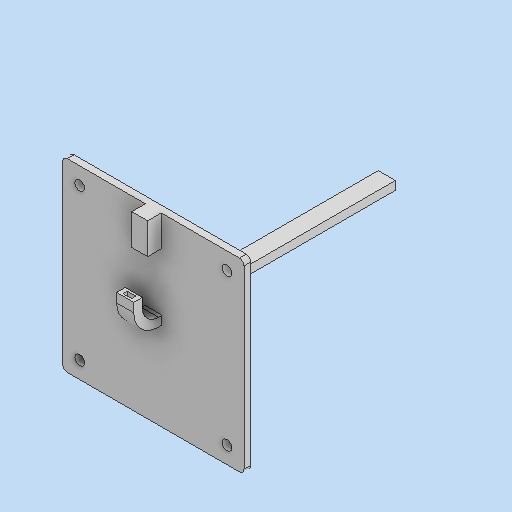
# Autodesk Inventor part: ProbeAntennaDummy
Saved by Autodesk Inventor 2023.2 (Build 272271000, 271)
## iProperties
Created: 2024-02-15
Part Number: ProbeAntennaDummy
Material: Generisch
Document SubType Name: Modeling
Designer: Nils Bade
Density: 1 g/cm^3
Appearance: Vorgabe
Description: Dummy
Auf Bestellliste: True
Author: Nils Bade
Autodesk Inventor part; units mm, degrees
sketch "S-Basis" plane through (0, 0, 0) normal (0, 0, 1) x (1, 0, 0)
  line L0 (0, 57.19) -> (0, -57.19) construction
  line L1 (-56, 0) -> (56, 0) construction
  line L2 (1.8795, -0.94) -> (1.8795, 0.94)
  line L3 (1.8795, 0.94) -> (-1.8795, 0.94)
  line L4 (-1.8795, 0.94) -> (-1.8795, -0.94)
  line L5 (-1.8795, -0.94) -> (1.8795, -0.94)
  line L6 (1.8795, -0.94) -> (-1.8795, 0.94) construction
  line L7 (1.8795, 0.94) -> (-1.8795, -0.94) construction
  line L8 (-40, 40.85) -> (40, 40.85)
  line L9 (40, 40.85) -> (40, -40.85)
  line L10 (40, -40.85) -> (-40, -40.85)
  line L11 (-40, -40.85) -> (-40, 40.85)
  line L12 (-40, 40.85) -> (40, -40.85) construction
  line L13 (40, 40.85) -> (-40, -40.85) construction
  line L14 (-40, 33.35) -> (40, 33.35) construction
  circle A0 centre (0, 33.35) radius 2.5 construction
  line L15 (-40, 13.03) -> (40, 13.03) construction
  line L16 (-3.7747, 1.8879) -> (3.7747, 1.8879)
  line L17 (3.7747, 1.8879) -> (3.7747, -1.8879)
  line L18 (3.7747, -1.8879) -> (-3.7747, -1.8879)
  line L19 (-3.7747, -1.8879) -> (-3.7747, 1.8879)
  line L20 (-3.7747, 1.8879) -> (3.7747, -1.8879) construction
  line L21 (3.7747, 1.8879) -> (-3.7747, -1.8879) construction
  circle A1 centre (-32.5, 33.35) radius 2.15
  circle A2 centre (32.5, 33.35) radius 2.15
  circle A3 centre (-32.5, -33.35) radius 2.15
  circle A4 centre (32.5, -33.35) radius 2.15
  line L22 (-3.5, 40.85) -> (3.5, 40.85)
  line L23 (3.5, 40.85) -> (3.5, 27.1517)
  line L24 (3.5, 27.1517) -> (-3.5, 27.1517)
  line L25 (-3.5, 27.1517) -> (-3.5, 40.85)
  point P0 (0, 0)
  point P1 (0, 40.85)
  dimension "d0" = 81.7
  dimension "d1" = 80
  dimension "d2" = 3.759
  dimension "d3" = 1.88
  dimension "d4" = 7.5
  dimension "d5" = 5
  dimension "d6" = 20.32
  dimension "d7" = 4.3
  dimension "d8" = 32.5
  dimension "d9" = 4.3
  dimension "d10" = 32.5
  dimension "d11" = 7.5
  dimension "d23" = 7
  constraints: 48 end point, 8 midpoint, 8 parallel, 7 point on line, 6 perpendicular, 5 centre point, 4 horizontal, 2 symmetric about line, 2 other
  measures "d0" distance of L8.end L9.end
  measures "d1" distance of L8.start L8.end
  measures "d2" distance of L2.end L3.end
  measures "d3" distance of L2.start L2.end
  measures "d4" distance between parallel lines of L14 L8
  measures "d5" diameter of A0
  measures "d6" distance from line of L15 A0.centre
  measures "d7" diameter of A1
  measures "d8" distance from line of L0 A1.centre
  measures "d9" diameter of A3
  measures "d10" distance from line of L0 A3.centre
  measures "d11" distance from line of L10 A3.centre
  measures "d23" distance of L23.end L24.end
ref_plane "Anschlussebene-Übergang" through (-40, 13.03, 0) normal (0, 1, 0) x (1, 0, 0)
extrude "Ex-Base1" add sketch "S-Basis" against normal blind 3 contours L8 L25 L24 L23 L9 L10 L11 | L8 L23 L24 L25 | L16 L17 L18 L19
extrude "Ex-Probe" add sketch "S-Basis" against normal blind 103 contours L16 L17 L18 L19
sketch "Skizze2" plane through (0, 0, 0) normal (1, 0, 0) x (0, 1, 0)
  line L0 (13.03, 14.8668) -> (13.03, -2.4778) projected
  line L1 (0, 14.8668) -> (0, -2.4778) projected
  line L2 (-4.8428, 0) -> (16.0088, 0) projected
  line L3 (13.03, 10.525) -> (9, 10.525)
  line L4 (0, 0) -> (0, 1.525)
  arc A0 (9, 10.525) -> (0, 1.525) centre (9, 1.525) ccw
  dimension "d18" = 10.525
  dimension "d19" = 9
  constraints: 4 end point, 2 point on circle, 2 point on line, 2 tangent, 1 centre point, 1 horizontal
  measures "d18" distance between parallel lines of L2 L3
  measures "d19" radius of A0
sweep "Sweep-Anschluss" add profiles "S-Basis" path "Skizze2" path curves L4 A0 L3 contours L16 L17 L18 L19
fillet "Rundung1" radius 2 4 edges at (40, -40.85, -1.5) (-40, -40.85, -1.5) (40, 40.85, -1.5) (-40, 40.85, -1.5)
ref_plane "RWG-X" through (1.8795, 9, 10.525) normal (0, 0, -1) x (-1, 0, 0)
ref_plane "RWG-Y" through (0, 9, 9.585) normal (1, 0, 0) x (0, 0, -1)
extrude "Extrusion3" add sketch "S-Basis" along normal blind 6 contours L8 L23 L24 L25
equation "\"d10\" = d8"
equation "\"d11\" = d4"
